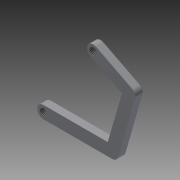
# Autodesk Inventor part: Servo_Arm_Hook_F_new
Saved by Autodesk Inventor 2015 SP2 (Build 190223200, 223)
## iProperties
Created: 2016-09-15
Part Number: Servo_Arm_Hook_F_new
Material: Generic
Document SubType Name: Modeling
Designer: jm799
Density: 1 g/cm^3
Appearance: Default
Author: jm799
Autodesk Inventor part; units mm, degrees
ref_plane "YZ Plane" through (0, 0, 0) normal (1, 0, 0) x (0, 1, 0)
ref_plane "XZ Plane" through (0, 0, 0) normal (0, 1, 0) x (-1, 0, 0)
ref_plane "XY Plane" through (0, 0, 0) normal (0, 0, 1) x (1, 0, 0)
sketch "Sketch1" plane through (0, 0, 0) normal (0, 1, 0) x (-1, 0, 0)
  circle A0 centre (0, 0) radius 2.5
  circle A1 centre (-27.7848, -0.0003) radius 2.5
  circle A2 centre (-34.6699, 23.8458) radius 2.5
  circle A3 centre (-20.1174, 31.2789) radius 2.5
  line L0 (-32.1699, 23.8458) -> (-25.2848, -0.0003)
  line L1 (-37.1699, 23.8458) -> (-30.1893, -0.6845)
  line L2 (-27.9447, 2.4946) -> (-0.0005, 2.5)
  line L3 (-0.0005, -2.5) -> (-27.7848, -2.5003)
  line L4 (-19.1471, 28.9749) -> (-33.5318, 21.6199)
  arc A4 (-33.5318, 21.6199) -> (-35.8061, 26.0727) centre (-34.6699, 23.8458) ccw
  line L5 (-21.4171, 33.4145) -> (-35.8061, 26.0727)
  dimension "d0" = 5
  dimension "d1" = 5
  dimension "d2" = 5
  dimension "d3" = 5
  constraints: 14 point on circle, 12 end point, 6 tangent, 5 centre point, 2 coincident
  measures "d0" diameter of A0
  measures "d1" diameter of A1
  measures "d2" diameter of A2
  measures "d3" diameter of A3
extrude "Extrusion1" add sketch "Sketch1" along normal blind 3 contours A0 | A0 L3 A1 L0 L2 | L0 A1 L1 A2 L4 | A1 L0 | L4 A2 L0 | L0 A2 L5 A3 L4 | A1 L0 | A2 L1 | A3 picked at (-35.4421, 23.1763)
sketch "Sketch2" plane through (0, 0, 0) normal (0, -1, 0) x (1, 0, 0)
  circle A0 centre (0, 0) radius 1.4
  dimension "d6" = 2.8
  constraints: 1 centre point, 1 coincident
  measures "d6" diameter of A0
extrude "Extrusion2" cut sketch "Sketch2" against normal blind 8
thread "Thread2" size "M3x0.5" class "6H" standard "ANSI Metric M Profile" full length
sketch "Sketch3" plane through (0, 0, 0) normal (0, -1, 0) x (1, 0, 0)
  arc A0 (21.4171, 33.4145) -> (19.1471, 28.9749) centre (20.1174, 31.2789) ccw projected
  circle A1 centre (20.1174, 31.2789) radius 1.5
  point P0 (0, 0)
  dimension "d13" = 3
  constraints: 1 centre point, 1 coincident
  measures "d13" diameter of A1
extrude "Extrusion3" cut sketch "Sketch3" against normal blind 10
thread "Thread3" size "M3x0.5" class "6H" standard "ANSI Metric M Profile" full length
body "Solid1"
